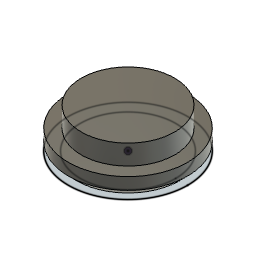
nixie_rohr_abdeckung_24x30 v2 (Autodesk Fusion 360 design; units mm, degrees)
Autodesk Fusion 360 part; units mm, degrees
sketch "Skizze1" plane through (0, 0, 0) normal (0, 1, 0) x (1, 0, 0)
  circle A0 centre (0, 0) radius 12
  circle A1 centre (0, 0) radius 15
  dimension "d1" = 24
  dimension "d2" = 30
  constraint coincident A0.centre A1.centre
  constraint concentric A0 A1
  measures "d1" diameter of A0
  measures "d2" diameter of A1
extrude "Extrusion1" add sketch "Skizze1" along normal blind 5
extrude "Extrusion2" add sketch "Skizze1" along normal blind 10 contours A0
chamfer "Fase1" distance 2 angle 45 1 edges at (-13.9849, 0, 5.4242)
sketch "Skizze2" plane through (0, 10, 0) normal (0, 1, 0) x (-1, 0, 0)
  circle A0 centre (0, 0) radius 12
  circle A1 centre (0, 0) radius 12
  circle A2 centre (0, 0) radius 11.75
  dimension "d8" = 23.5
  constraint coincident A0.centre A1.centre
  measures "d8" diameter of A2
extrude "Extrusion3" cut sketch "Skizze2" against normal blind 5
